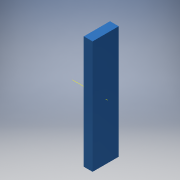
# Autodesk Inventor part: TCD1304AP
Saved by Autodesk Inventor 2017 (Build 210142000, 142)
## iProperties
Created: 2017-01-24
Part Number: TCD1304AP
Material: Glass
Document SubType Name: Modeling
Designer: vmigu
Density: 2.18 g/cm^3
Appearance: Cyan
Author: vmigu
Autodesk Inventor part; units mm, degrees
ref_plane "YZ Plane" through (0, 0, 0) normal (1, 0, 0) x (0, 1, 0)
ref_plane "XZ Plane" through (0, 0, 0) normal (0, 1, 0) x (-1, 0, 0)
ref_plane "XY Plane" through (0, 0, 0) normal (0, 0, 1) x (1, 0, 0)
sketch "Sketch1" plane through (0, 0, 0) normal (1, 0, 0) x (0, 1, 0)
  line L0 (4.825, 20.8) -> (-4.825, 20.8)
  line L1 (-4.825, 20.8) -> (-4.825, -20.8)
  line L2 (-4.825, -20.8) -> (4.825, -20.8)
  line L3 (4.825, -20.8) -> (4.825, 20.8)
  line L4 (4.825, 20.8) -> (-4.825, -20.8) construction
  line L5 (-4.825, 20.8) -> (4.825, -20.8) construction
  point P0 (0, 0)
  dimension "d0" = 9.65
  dimension "d1" = 41.6
  constraints: 12 end point, 2 midpoint, 2 parallel, 1 horizontal, 1 perpendicular
  measures "d0" distance of L2.end L1.end
  measures "d1" distance of L1.end L0.end
extrude "Extrusion1" add sketch "Sketch1" along normal blind 3.22
sketch "Sketch2" plane through (0, 0, 0) normal (-1, 0, 0) x (0, 0, 1)
  line L0 (-14.55, 0.5) -> (14.55, 0.5)
  line L1 (14.55, 0.5) -> (14.55, -0.5)
  line L2 (14.55, -0.5) -> (-14.55, -0.5)
  line L3 (-14.55, -0.5) -> (-14.55, 0.5)
  line L4 (-14.55, 0.5) -> (14.55, -0.5) construction
  line L5 (14.55, 0.5) -> (-14.55, -0.5) construction
  point P0 (0, 0)
  dimension "d4" = 29.1
  dimension "d5" = 1
  constraints: 12 end point, 2 midpoint, 2 parallel, 1 horizontal, 1 perpendicular
  measures "d4" distance of L1.end L2.end
  measures "d5" distance of L0.end L1.end
extrude "Extrusion2" cut sketch "Sketch2" against normal blind 1.52
chamfer "Chamfer1" distance 1.52 angle 45 4 edges at (0, 0.5, 0) (0, 0, -14.55) (0, -0.5, 0) (0, 0, 14.55)
sketch "Sketch3" plane through (1.52, 0, 0) normal (-1, 0, 0) x (0, 0, 1)
  point P0 (0, 0)
body "Solid1"
